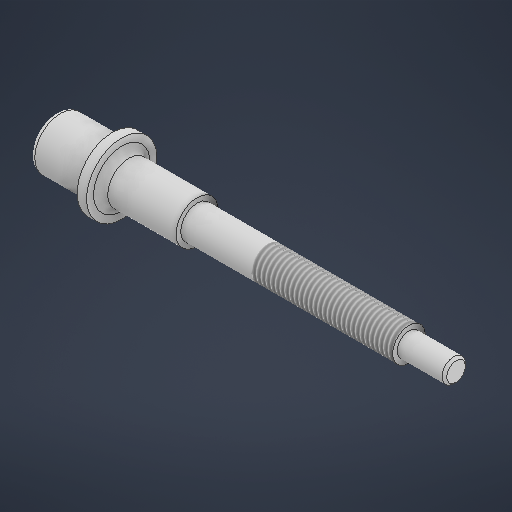
# Autodesk Inventor part: Part6
Saved by Autodesk Inventor 2026 (Build 300175050, 175E)
## iProperties
Created: 2026-03-26
Part Number: Part6
Material: Generic
Document SubType Name: Modeling
Designer: Administrator
Density: 1 g/cm^3
Appearance: Default
Author: Administrator
Autodesk Inventor part; units mm, degrees
ref_plane "YZ Plane" through (0, 0, 0) normal (1, 0, 0) x (0, 1, 0)
ref_plane "XZ Plane" through (0, 0, 0) normal (0, 1, 0) x (-1, 0, 0)
ref_plane "XY Plane" through (0, 0, 0) normal (0, 0, 1) x (1, 0, 0)
sketch "Sketch1" plane through (0, 0, 0) normal (0, 0, 1) x (1, 0, 0)
  line L0 (0, 0) -> (170, 0)
  line L1 (170, 0) -> (170, 5)
  line L2 (170, 5) -> (150, 5)
  line L3 (150, 5) -> (150, 7)
  line L4 (150, 7) -> (90, 7)
  line L5 (90, 7) -> (60, 7)
  line L6 (60, 7) -> (60, 9)
  line L7 (60, 9) -> (28, 9)
  line L8 (28, 9) -> (28, 15)
  line L9 (28, 15) -> (24, 15)
  line L10 (24, 15) -> (24, 11)
  line L11 (24, 11) -> (0, 11)
  line L12 (0, 11) -> (0, 0)
  dimension "d0" = 170
  dimension "d1" = 10
  dimension "d2" = 14
  dimension "d3" = 18
  dimension "d4" = 30
  dimension "d5" = 22
  dimension "d6" = 24
  dimension "d7" = 4
  dimension "d8" = 32
  dimension "d9" = 60
  dimension "d10" = 30
  constraints: 26 end point, 9 perpendicular, 2 vertical, 1 horizontal, 1 point on line
  measures "d0" distance of L0.start L0.end
  measures "d1" diameter of L2 L0
  measures "d2" diameter of L4 L0
  measures "d3" diameter of L7 L0
  measures "d4" diameter of L9 L0
  measures "d5" diameter of L11 L0
  measures "d6" distance of L10.end L11.end
  measures "d7" distance of L8.end L9.end
  measures "d8" distance of L6.end L7.end
  measures "d9" distance of L3.end L4.end
  measures "d10" distance of L4.end L5.end
revolve "Revolution1" add sketch "Sketch1" angle 360 about axis through (0, 0, 0) along (1, 0, 0)
thread "Thread1" size "M14x2" class "6g" standard "ANSI Metric M Profile" length 60
fillet "Fillet1" radius 3 1 edges at (28, -9, 0)
fillet "Fillet2" radius 2 1 edges at (0, -11, 0)
chamfer "Chamfer1" distance 1 angle 45 1 edges at (170, -5, 0)
body "Solid1"
